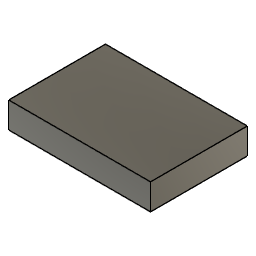
MotorContainerRaiser v1 (Autodesk Fusion 360 design; units mm, degrees)
Autodesk Fusion 360 part; units mm, degrees
sketch "Sketch1" plane through (0, 0, 0) normal (0, 0, 1) x (1, 0, 0)
  line L0 (0, 0) -> (76.2, 0)
  line L1 (76.2, 0) -> (76.2, 51.9938)
  line L2 (76.2, 51.9938) -> (0, 51.9938)
  line L3 (0, 51.9938) -> (0, 0)
  dimension "d3" = 76.2
  dimension "d4" = 51.9938
  constraint horizontal L0
  constraint vertical L1
  constraint horizontal L2
  constraint vertical L3
  constraint coincident L0.start L3.end
  measures "d3" distance of L0.start L0.end
  measures "d4" distance of L0.start L2.end
extrude "Extrude1" add sketch "Sketch1" along normal blind 13.97
equation "length = 3 in"
equation "Width = 2.047 in"
equation "d3 = length"
equation "d4 = Width"
equation "height = 0.55 in"
equation "d6 = height"
